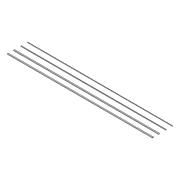
# Autodesk Inventor part: WAVEGUIDES
Saved by Autodesk Inventor 2019.4 (Build 234330000, 330)
## iProperties
Created: 2021-03-16
Part Number: WAVEGUIDES
Material: Generic
Document SubType Name: Modeling
Designer: diederichbenedict
Density: 1 g/cm^3
Appearance: Default
Author: diederichbenedict
Autodesk Inventor part; units mm, degrees
ref_plane "YZ Plane" through (0, 0, 0) normal (1, 0, 0) x (0, 1, 0)
ref_plane "XZ Plane" through (0, 0, 0) normal (0, 1, 0) x (-1, 0, 0)
ref_plane "XY Plane" through (0, 0, 0) normal (0, 0, 1) x (1, 0, 0)
sketch "Sketch1" plane through (0, 0, 0) normal (0, 1, 0) x (-1, 0, 0)
  line L0 (0, 0) -> (70, 0)
  line L1 (70, 0) -> (70, -0.5)
  line L2 (70, -0.5) -> (0, -0.5)
  line L3 (0, -0.5) -> (0, 0)
  line L4 (70, -3.5) -> (0, -3.5)
  line L5 (0, -3.5) -> (0, -3.7)
  line L6 (0, -3.7) -> (70, -3.7)
  line L7 (70, -3.7) -> (70, -3.5)
  line L8 (70, -6.7) -> (0, -6.7)
  line L9 (0, -6.7) -> (0, -6.8)
  line L10 (0, -6.8) -> (70, -6.8)
  line L11 (70, -6.8) -> (70, -6.7)
  line L12 (0, 3) -> (70, 3)
  line L13 (70, 3) -> (70, 2.5)
  line L14 (70, 2.5) -> (0, 2.5)
  line L15 (0, 2.5) -> (0, 3)
  point P0 (70, -4.8229)
  dimension "d0" = 70
  dimension "d1" = 0.5
  dimension "d2" = 70
  dimension "d3" = 0.2
  dimension "d4" = 3
  dimension "d5" = 70
  dimension "d6" = 0.1
  dimension "d7" = 3
  dimension "d8" = 0
  dimension "d9" = 70
  dimension "d10" = 0.5
  dimension "d11" = 3
  dimension "d12" = 0
  constraints: 32 end point, 8 parallel, 4 horizontal, 4 perpendicular, 2 point on line
  measures "d0" distance of L1.end L2.end
  measures "d1" distance of L0.end L1.end
  measures "d2" distance of L6.end L5.end
  measures "d3" distance of L5.end L4.end
  measures "d4" distance between parallel lines of L2 L4
  measures "d5" distance of L10.end L9.end
  measures "d6" distance of L9.end L8.end
  measures "d7" distance between parallel lines of L6 L8
  measures "d8" distance between parallel lines of L9 L3
  measures "d9" distance of L13.end L14.end
  measures "d10" distance of L13.start L13.end
  measures "d11" distance of L2.end L14.end
  measures "d12" horizontal distance of L0.start L14.end
extrude "Extrusion1" add sketch "Sketch1" along normal blind 0.3
body "Solid1"
